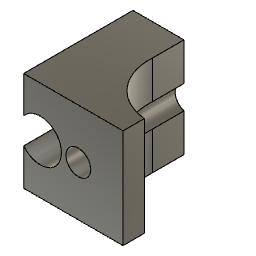
pied laser v1 (Autodesk Fusion 360 design; units mm, degrees)
Autodesk Fusion 360 part; units mm, degrees
sketch "Sketch1" plane through (0, 0, 0) normal (0, 1, 0) x (1, 0, 0)
  line L0 (0, 0) -> (20, 0)
  line L1 (20, 0) -> (20, 20)
  line L2 (20, 20) -> (0, 20)
  line L3 (0, 20) -> (0, 0)
  dimension "d1" = 20
  dimension "d2" = 20
  constraint horizontal L0
  constraint vertical L1
  constraint horizontal L2
  constraint vertical L3
  constraint coincident L0.start L3.end
  measures "d1" distance of L0.start L0.end
  measures "d2" distance of L0.start L2.end
extrude "Extrude1" add sketch "Sketch1" along normal blind 22
sketch "Sketch2" plane through (0, 0, 0) normal (0, 0, 1) x (-1, 0, 0)
  line L0 (0, 0) -> (-20, 0)
  line L1 (-20, 0) -> (-20, -22)
  line L2 (-20, -22) -> (0, -22)
  line L3 (0, -22) -> (0, 0)
  circle A0 centre (-21, -15) radius 10.75
  dimension "d5" = 21.5
  measures "d5" diameter of A0
extrude "Extrude2" cut sketch "Sketch2" against normal blind 33 contours L1 L2 A0 picked at (-19.4784, -10.2857)
sketch "Sketch3" plane through (0, 0, 0) normal (0, -1, 0) x (1, 0, 0)
  line L0 (0, 0) -> (0, -20)
  line L1 (0, -20) -> (20, -20)
  line L2 (20, -20) -> (20, 0)
  line L3 (20, 0) -> (0, 0)
  circle A0 centre (3.3477, -10) radius 2
  circle A1 centre (3.3477, -10) radius 4.25
  circle A2 centre (11, -10) radius 2.5
  dimension "d8" = 4
  dimension "d9" = 8.5
  dimension "d10" = 5
  constraint concentric A0 A1
  measures "d8" diameter of A0
  measures "d9" diameter of A1
  measures "d10" diameter of A2
extrude "Extrude3" cut sketch "Sketch3" against normal blind 33 contours A0 | A2
extrude "Extrude4" cut sketch "Sketch3" against normal blind 18 contours L0 A1 picked at (0.4492, -10)
sketch "Sketch4" plane through (0, 0, 0) normal (0, 0, 1) x (-1, 0, 0)
  arc A0 (-12.8414, -22) -> (-20, -4.2966) centre (-21, -15) ccw
  line L0 (-12.8414, -22) -> (0, -22)
  line L1 (0, -22) -> (0, 0)
  line L2 (0, 0) -> (-20, 0)
  line L3 (-20, 0) -> (-20, -4.2966)
  line L4 (-10.3695, -13.4018) -> (-17, -13.4018)
  line L5 (-17, -13.4018) -> (-17, -25)
  line L6 (-17, -25) -> (-10.3695, -25)
  line L7 (-10.3695, -25) -> (-10.3695, -13.4018)
  constraint horizontal L4
  constraint vertical L5
  constraint horizontal L6
  constraint vertical L7
  constraint coincident A0 L4.start
extrude "Extrude5" cut sketch "Sketch4" against normal blind 33 contours A0 L0 L7
move_face "OffsetFaces1" offset -0.1 2 faces at (10.3695, 20.1994, -5.0539) (10.3695, 20.1994, -14.9461)
